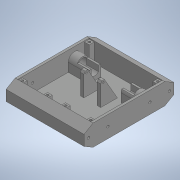
# Autodesk Inventor part: HexBody
Saved by Autodesk Inventor 2020 (Build 240168000, 168)
## iProperties
Created: 2023-12-19
Part Number: HexBody
Material: H TPU
Document SubType Name: Modeling
Designer: smz3rm
Density: 0.941117 g/cm^3
Appearance: Generic(1)
Mass: 192.809 g
Surface Area: 757.089 cm^2
Volume: 204.872 cm^3
BaseThickness: 3.000 mm
TopThickness: 1.778 mm
SideThickness: 4.000 mm
BodyWidth: 130.000 mm
BodyLength: 150.000 mm
BodyHeight: 35.000 mm
DriveMotorHeight: 17.500 mm
WheelWidth: 13.000 mm
WheelGrooveWidth: 4.000 mm
WheelGrooveDia: 15.400 mm
WheelDia: 38.500 mm
WheelPulleyDia: 2.000 mm
M3ScrewInsertBrim: 8.000 mm
M3ScrewDia: 3.100 mm
M3ScrewHeadDia: 6.100 mm
M3ScrewInsertDia: 4.000 mm
M3ScrewInsertDepth: 7.000 mm
DriveMotorOffset: 40.000 mm
DriveMotorHoleDia: 4.200 mm
M3ScrewHeadDepth: 2.200 mm
M3ScrewHeadTaper: -32.50 deg
WheeGuardlSlotWidth: 20.000 mm
WheelGuardScrewOffset: 7.000 mm
FlipperLength: 90.000 mm
FlipperThickness: 4.000 mm
FlipperWidth: 20.000 mm
WheelSpokes: 5.000 ul
FlipperRodDia: 2.000 mm
Author: smz3rm
Autodesk Inventor part; units mm, degrees
ref_plane "XZ Plane" through (0, 0, 0) normal (0, 1, 0) x (-1, 0, 0)
ref_plane "XY Plane" through (0, 0, 0) normal (0, 0, 1) x (1, 0, 0)
sketch "Sketch1" plane through (0, 0, 0) normal (1, 0, 0) x (0, 1, 0)
  line L0 (-17.5, 75) -> (17.5, 75)
  line L1 (17.5, 75) -> (17.5, -75)
  line L2 (17.5, -75) -> (-17.5, -75)
  line L3 (-17.5, -75) -> (-17.5, 75)
  line L4 (-17.5, 75) -> (17.5, -75) construction
  line L5 (17.5, 75) -> (-17.5, -75) construction
  line L6 (-24.5, 0) -> (24.5, 0) projected
  line L7 (0, -105) -> (0, 105) projected
  line L8 (8.75, -75) -> (-8.75, -75)
  line L9 (-8.75, -75) -> (-17.5, -59.8446)
  line L10 (-17.5, -59.8446) -> (-8.75, -44.6891)
  line L11 (-8.75, -44.6891) -> (8.75, -44.6891)
  line L12 (8.75, -44.6891) -> (17.5, -59.8446)
  line L13 (17.5, -59.8446) -> (8.75, -75)
  line L14 (-8.75, 75) -> (-17.5, 59.8446)
  line L15 (17.5, 59.8446) -> (8.75, 75)
  point P0 (0, 0)
  point P1 (0, -59.8446)
  dimension "d0" = 35
  dimension "d1" = 150
  dimension "d25" = 15.1554
  constraints: 28 end point, 4 point on line, 4 symmetric about line, 2 midpoint, 2 parallel, 1 horizontal, 1 perpendicular, 13 other
  measures "d0" distance of L1.end L2.end
  measures "d1" distance of L0.end L1.end
  measures "d25" distance from line of point (0, -59.845) L2
extrude "Extrusion1" add sketch "Sketch1" along normal mid plane 130 contours L0 L7 L6 L3 L14 | L0 L15 L1 L6 L7 | L6 L7 L11 L10 L3 | L6 L1 L12 L11 L7 | L10 L11 L7 L2 L9 | L11 L12 L13 L2 L7
sketch "Sketch2" plane through (-65, 17.5, 60.2776) normal (0, 1, 0) x (1, 0, 0)
  line L0 (130, 120.1221) -> (130, 0.433) projected
  line L1 (0, 0.433) -> (0, 120.1221) projected
  line L2 (126, 120.1221) -> (4, 120.1221)
  line L3 (4, 120.1221) -> (4, 0.433)
  line L4 (4, 0.433) -> (126, 0.433)
  line L5 (126, 0.433) -> (126, 120.1221)
  line L6 (126, 120.1221) -> (4, 0.433) construction
  line L7 (4, 120.1221) -> (126, 0.433) construction
  line L8 (0, 0.433) -> (130, 0.433) projected
  line L9 (0, 120.1221) -> (130, 120.1221) projected
  point P0 (65, 60.2776)
  dimension "d4" = 4
  constraints: 12 end point, 2 midpoint, 2 parallel, 1 horizontal, 1 perpendicular, 1 point on line
  measures "d4" distance between parallel lines of L1 L3
extrude "Extrusion2" cut sketch "Sketch2" against normal blind 32 contours L5 L4 L3 L2
sketch "Sketch3" plane through (-65, -14.5, 60.2776) normal (0, 1, 0) x (1, 0, 0)
  line L0 (4, 0.433) -> (4, 120.1221) projected
  line L1 (126, 0.433) -> (4, 0.433) projected
  line L2 (126, 120.1221) -> (126, 0.433) projected
  line L3 (4, 120.1221) -> (126, 120.1221) projected
  line L4 (4, 0.433) -> (4, 120.1221) projected
  line L5 (126, 120.1221) -> (126, 0.433) projected
  line L6 (130, 120.1221) -> (130, 0.433) projected
  line L7 (0, 0.433) -> (0, 120.1221) projected
  line L8 (4, 120.1221) -> (12, 120.1221)
  line L9 (12, 120.1221) -> (12, 112.1221)
  line L10 (12, 112.1221) -> (4, 112.1221)
  line L11 (4, 112.1221) -> (4, 120.1221)
  line L12 (-26, 60.2776) -> (156, 60.2776) projected
  line L13 (65, 165.2776) -> (65, -44.7224) projected
  line L14 (118, 120.1221) -> (118, 112.1221)
  line L15 (118, 112.1221) -> (126, 112.1221)
  line L16 (12, 0.433) -> (12, 8.433)
  line L17 (12, 8.433) -> (4, 8.433)
  line L18 (118, 0.433) -> (118, 8.433)
  line L19 (118, 8.433) -> (126, 8.433)
  line L20 (0, 120.1221) -> (4, 120.1221) projected
  line L21 (0, 0.433) -> (4, 0.433) projected
  line L22 (126, 0.433) -> (130, 0.433) projected
  line L23 (126, 120.1221) -> (130, 120.1221) projected
  point P0 (65, 60.2776)
  point P1 (12, 0.433)
  point P2 (4, 112.1221)
  point P3 (126, 8.433)
  point P4 (118, 0.433)
  dimension "d8" = 8
  constraints: 20 end point, 9 symmetric about line, 2 parallel, 2 perpendicular, 1 horizontal
  measures "d8" distance of L9.end L10.end
extrude "Extrusion3" add sketch "Sketch3" along normal blind 30.222 contours L0 L17 L16 L1 | L0 L3 L9 L10 | L18 L19 L2 L1 | L15 L14 L3 L2
sketch "Sketch4" plane through (-61, 17.5, 59.8446) normal (1, 0, 0) x (0, 0, -1)
  circle A0 centre (94.8446, -17.5) radius 8.25
  line L0 (119.6891, -35) -> (0, -35) projected
  line L1 (134.8446, -8.75) -> (134.8446, -26.25) projected
  circle A1 centre (94.8446, -17.5) radius 10.25
  line L2 (84.5946, -17.5) -> (84.5946, -32)
  line L3 (8, -32) -> (111.6891, -32) projected
  line L4 (105.0946, -17.5) -> (105.0946, -32)
  point P0 (59.8446, -17.5)
  dimension "d12" = 16.5
  dimension "d13" = 17.5
  dimension "d14" = 40
  dimension "d15" = 2
  constraints: 4 end point, 2 centre point, 2 point on circle, 2 point on line, 2 tangent, 2 vertical, 1 coincident
  measures "d12" diameter of A0
  measures "d13" distance from line of L0 A0.centre
  measures "d14" distance from line of L1 A0.centre
  measures "d15" radial gap between concentric circles of A0 A1
extrude "Extrusion4" add sketch "Sketch4" along normal blind 14
sketch "Sketch5" plane through (-47, 17.5, 59.8446) normal (1, 0, 0) x (0, 0, -1)
  circle A0 centre (94.8446, -17.5) radius 8.25 projected
  circle A1 centre (94.8446, -17.5) radius 7.75
  line L0 (105.0946, -32) -> (105.0946, -17.5) projected
  arc A2 (105.0946, -17.5) -> (84.5946, -17.5) centre (94.8446, -17.5) ccw projected
  line L1 (84.5946, -17.5) -> (84.5946, -32) projected
  line L2 (105.0946, -32) -> (84.5946, -32) projected
  circle A3 centre (94.8446, -17.5) radius 8.25 projected
  line L3 (88.7446, -12.7196) -> (85.7776, -12.7196)
  arc A4 (105.0946, -17.5) -> (84.5946, -17.5) centre (94.8446, -17.5) ccw projected
  line L4 (88.7446, -12.7196) -> (88.7446, -32)
  line L5 (105.0946, -32) -> (84.5946, -32) projected
  line L6 (100.9446, -12.7196) -> (103.9115, -12.7196)
  line L7 (100.9446, -12.7196) -> (100.9446, -32)
  point P0 (59.8446, -17.5)
  point P1 (88.7446, -22.2804)
  point P2 (85.7776, -12.7196)
  point P3 (100.9446, -22.2804)
  dimension "d18" = 15.5
  dimension "d19" = 12.2
  constraints: 8 end point, 4 point on circle, 2 horizontal, 2 perpendicular, 2 point on line, 1 centre point, 1 coincident, 1 parallel
  measures "d18" diameter of A1
  measures "d19" distance between parallel lines of L7 L4
extrude "Extrusion5" add sketch "Sketch5" along normal blind 20 contours A0 L7 A1 L6 | A0 L6 A2 L0 L2 L7 | L7 L2 L4 A0 | A0 L4 A1 L7 | L3 A1 L4 A0 | A0 L4 L2 L1 A2 L3 | A1 L7 | L4 A1
sketch "Sketch6" plane through (-61, 0, -35) normal (1, 0, 0) x (0, 0, -1)
  circle A0 centre (0, 0) radius 2.1
  point P0 (-35, 0)
  dimension "d22" = 4.2
  constraints: 1 centre point
  measures "d22" diameter of A0
extrude "Extrusion6" cut sketch "Sketch6" against normal through all
mirror "Mirror1" about plane through (0, 0, 0) normal (1, 0, 0) of "Extrusion4", "Extrusion5", "Extrusion6"
sketch "Sketch7" plane through (-65, 0, 0) normal (-1, 0, 0) x (0, 0, 1)
  line L0 (-105, 0) -> (105, 0) projected
  circle A0 centre (35, 0) radius 2
  line L1 (75, -8.75) -> (75, 8.75) projected
  point P0 (0, 0)
  dimension "d26" = 4
  dimension "d27" = 40
  constraints: 1 centre point, 1 point on line
  measures "d26" diameter of A0
  measures "d27" distance from line of L1 A0.centre
extrude "Extrusion7" cut sketch "Sketch7" against normal up to surface (4 mm away)
mirror "Mirror2" about plane through (0, 0, 0) normal (1, 0, 0) of "Extrusion7"
sketch "Sketch9" plane through (-65, 0, 0) normal (-1, 0, 0) x (0, 0, 1)
  line L0 (-59.8446, 17.5) -> (-59.8446, 15.722) projected
  line L1 (-59.8446, -17.5) -> (-59.8446, 17.5)
  line L2 (-75, -8.75) -> (-75, 8.75) projected
  line L3 (-75, 0) -> (-59.8446, 0)
  line L4 (-59.8446, -14.5) -> (-59.8446, 15.722) projected
  circle A0 centre (-67.4223, 0) radius 2
  line L5 (0, -24.5) -> (0, 24.5) projected
  circle A1 centre (67.4223, 0) radius 2
  point P0 (0, 0)
  dimension "d30" = 4
  constraints: 4 end point, 2 centre point, 2 midpoint, 1 perpendicular, 1 point on line, 1 symmetric about line, 1 vertical, 1 other
  measures "d30" diameter of A0
extrude "Extrusion8" cut sketch "Sketch9" against normal blind 7
mirror "Mirror3" about plane through (0, 0, 0) normal (1, 0, 0) of "Extrusion8"
ref_plane "Work Plane1" through (11, 0, 0) normal (1, 0, 0) x (0, 1, 0)
sketch "Sketch10" plane through (11, 0, 0) normal (1, 0, 0) x (0, 1, 0)
  line L0 (-14.5, 51.8446) -> (-14.5, -24.75) projected
  line L1 (-14.5, -0.9008) -> (23.05, -0.9008)
  line L2 (23.05, -0.9008) -> (23.05, -7.0496)
  line L3 (23.05, -7.0496) -> (-14.5, -28.7291)
  circle A0 centre (19.5, -5) radius 1.55
  line L4 (-8.75, -75) -> (8.75, -75) projected
  line L5 (17.5, -59.8446) -> (17.5, 59.8446) projected
  line L6 (-14.5, -24.75) -> (-14.5, -45.25) projected
  line L7 (-14.5, -24.75) -> (-14.5, 51.8446) projected
  line L8 (23.05, -7.0496) -> (19.5, -9.0992)
  line L9 (19.5, -9.0992) -> (15.95, -7.0496)
  line L10 (15.95, -7.0496) -> (15.95, -2.9504)
  line L11 (15.95, -2.9504) -> (19.5, -0.9008)
  line L12 (19.5, -0.9008) -> (23.05, -2.9504)
  line L13 (23.05, -2.9504) -> (23.05, -7.0496)
  point P0 (0, 0)
  point P1 (21.05, -5)
  point P2 (17.5, -10.2539)
  point P3 (17.5, -0.9008)
  dimension "d34" = 3.1
  dimension "d38" = 70
  dimension "d40" = 1.55
  dimension "d41" = 2
  dimension "d44" = 60
  dimension "d45" = 2
  constraints: 18 end point, 4 point on line, 1 coincident, 1 collinear, 1 horizontal, 1 horizontal alignment, 1 perpendicular, 15 other
  measures "d38" distance from line of L4 point (19.5, -5)
  measures "d40" distance of point (19.5, -5) point (21.05, -5)
  measures "d41" distance from line of L5 point (19.5, -5)
  measures "d44" angle of L0 L3
  measures "d45" distance from line of L13 point (21.05, -5)
extrude "Extrusion9" add sketch "Sketch10" along normal blind 6 contours L1 L5 L11 L10 L9 L3 L6 L0 | L1 L11 L5 | L12 L2 L3 L9 L5 L11 | L5 L9 L10 L11 | L5 L9 L3
mirror "Mirror4" about plane through (0, 0, 0) normal (1, 0, 0) of "Extrusion9"
sketch "Sketch12" plane through (-65, -14.5, 60.2776) normal (0, 1, 0) x (1, 0, 0)
  line L0 (48, 89.0067) -> (54, 89.0067) projected
  line L1 (54, 89.0067) -> (54, 61.1784) projected
  line L2 (54, 61.1784) -> (48, 61.1784) projected
  line L3 (48, 61.1784) -> (48, 89.0067) projected
  line L4 (76, 89.0067) -> (82, 89.0067) projected
  line L5 (82, 89.0067) -> (82, 61.1784) projected
  line L6 (82, 61.1784) -> (76, 61.1784) projected
  line L7 (76, 61.1784) -> (76, 89.0067) projected
  line L8 (126, 85.0276) -> (92, 85.0276) projected
  line L9 (92, 85.0276) -> (92, 105.5276) projected
  line L10 (92, 105.5276) -> (126, 105.5276) projected
  line L11 (126, 112.1221) -> (126, 105.5276) projected
  line L12 (126, 112.1221) -> (118, 112.1221) projected
  line L13 (118, 112.1221) -> (118, 120.1221) projected
  line L14 (12, 120.1221) -> (118, 120.1221) projected
  line L15 (12, 120.1221) -> (12, 112.1221) projected
  line L16 (12, 112.1221) -> (4, 112.1221) projected
  line L17 (4, 105.5276) -> (4, 112.1221) projected
  line L18 (4, 105.5276) -> (38, 105.5276) projected
  line L19 (38, 105.5276) -> (38, 85.0276) projected
  line L20 (38, 85.0276) -> (4, 85.0276) projected
  line L21 (4, 8.433) -> (4, 85.0276) projected
  line L22 (4, 8.433) -> (12, 8.433) projected
  line L23 (12, 8.433) -> (12, 0.433) projected
  line L24 (118, 0.433) -> (12, 0.433) projected
  line L25 (118, 0.433) -> (118, 8.433) projected
  line L26 (118, 8.433) -> (126, 8.433) projected
  line L27 (126, 85.0276) -> (126, 8.433) projected
  line L28 (54, 61.1784) -> (48, 61.1784) projected
  line L29 (54, 61.1784) -> (48, 61.1784) projected
  line L30 (82, 61.1784) -> (76, 61.1784) projected
  line L31 (76, 61.1784) -> (82, 61.1784) projected
  line L32 (118, 0.433) -> (12, 0.433) projected
  line L33 (54, 0.433) -> (46, 0.433)
  line L34 (46, 0.433) -> (46, 8.433)
  line L35 (46, 8.433) -> (54, 8.433)
  line L36 (54, 8.433) -> (54, 0.433)
  line L37 (65, 165.2776) -> (65, -44.7224) projected
  line L38 (84, 0.433) -> (84, 8.433)
  line L39 (84, 8.433) -> (76, 8.433)
  line L40 (76, 8.433) -> (76, 0.433)
  point P0 (65, 60.2776)
  dimension "d46" = 8
  constraints: 14 end point, 4 symmetric about line, 2 parallel, 2 perpendicular, 1 collinear, 1 horizontal, 1 point on line
  measures "d46" distance of L34.end L35.end
extrude "Extrusion10" add sketch "Sketch12" along normal blind 30.222 contours L24 L40 L39 L38 | L24 L34 L35 L36
sketch "Sketch13" plane through (-65, 15.722, 60.2776) normal (0, 1, 0) x (1, 0, 0)
  line L0 (4, 112.1221) -> (4, 120.1221) projected
  line L1 (4, 112.1221) -> (12, 112.1221) projected
  line L2 (12, 112.1221) -> (12, 120.1221) projected
  line L3 (4, 120.1221) -> (12, 120.1221) projected
  line L4 (118, 120.1221) -> (126, 120.1221) projected
  line L5 (118, 120.1221) -> (118, 112.1221) projected
  line L6 (118, 112.1221) -> (126, 112.1221) projected
  line L7 (126, 120.1221) -> (126, 112.1221) projected
  line L8 (126, 8.433) -> (126, 0.433) projected
  line L9 (126, 8.433) -> (118, 8.433) projected
  line L10 (118, 8.433) -> (118, 0.433) projected
  line L11 (126, 0.433) -> (118, 0.433) projected
  line L12 (84, 0.433) -> (76, 0.433) projected
  line L13 (84, 0.433) -> (84, 8.433) projected
  line L14 (84, 8.433) -> (76, 8.433) projected
  line L15 (76, 8.433) -> (76, 0.433) projected
  line L16 (54, 0.433) -> (54, 8.433) projected
  line L17 (54, 8.433) -> (46, 8.433) projected
  line L18 (46, 8.433) -> (46, 0.433) projected
  line L19 (54, 0.433) -> (46, 0.433) projected
  line L20 (12, 0.433) -> (4, 0.433) projected
  line L21 (12, 0.433) -> (12, 8.433) projected
  line L22 (12, 8.433) -> (4, 8.433) projected
  line L23 (4, 0.433) -> (4, 8.433) projected
  line L24 (4, 120.1221) -> (126, 120.1221) projected
  line L25 (4, 112.1221) -> (12, 112.1221) projected
  line L26 (4, 0.433) -> (4, 120.1221) projected
  line L27 (12, 120.1221) -> (12, 112.1221) projected
  line L28 (8, 120.1221) -> (8, 112.1221)
  line L29 (4, 116.1221) -> (12, 116.1221)
  line L30 (65, 165.2776) -> (65, -44.7224) projected
  line L31 (156, 60.2776) -> (-26, 60.2776) projected
  circle A0 centre (8, 116.1221) radius 2
  circle A1 centre (122, 116.1221) radius 2
  circle A2 centre (8, 4.433) radius 2
  circle A3 centre (122, 4.433) radius 2
  line L32 (50, 8.433) -> (50, 0.433)
  line L33 (46, 0.433) -> (46, 8.433) projected
  line L34 (46, 4.433) -> (54, 4.433)
  line L35 (54, 8.433) -> (54, 0.433) projected
  circle A4 centre (50, 4.433) radius 2
  circle A5 centre (80, 4.433) radius 2
  point P0 (65, 60.2776)
  dimension "d51" = 4
  dimension "d52" = 4
  constraints: 8 end point, 8 midpoint, 6 centre point, 4 symmetric about line, 2 point on line, 1 parallel, 1 perpendicular, 4 other
  measures "d51" diameter of A0
  measures "d52" diameter of A4
extrude "Extrusion11" cut sketch "Sketch13" against normal blind 7 contours A0 L28 L29 | L29 L28 A0 | L28 L29 A0 | L28 A0 L29 | A4 L32 L34 | L34 L32 A4 | A4 L34 L32 | L34 A4 L32 | A1 | A2 | A3 | A5
equation "\"d0\" = BodyHeight"
equation "\"d1\" = BodyLength"
equation "\"d2\" = BodyWidth"
equation "\"d4\" = SideThickness"
equation "\"d5\" = BodyHeight - BaseThickness"
equation "\"d8\" = M3ScrewInsertBrim"
equation "\"d10\" = -BaseThickness + BodyHeight - TopThickness"
equation "\"d13\" = DriveMotorHeight"
equation "\"d14\" = DriveMotorOffset"
equation "\"d22\" = DriveMotorHoleDia"
equation "\"d26\" = M3ScrewInsertDia"
equation "\"d27\" = DriveMotorOffset"
equation "\"d30\" = M3ScrewInsertDia"
equation "\"d31\" = M3ScrewInsertDepth"
equation "\"d34\" = M3ScrewDia"
equation "\"d38\" = FlipperMountOffset"
equation "\"d40\" = 0.5 * d34"
equation "\"d41\" = 0.5 * FlipperThickness"
equation "\"d42\" = FlipperMountThickness"
equation "\"d46\" = M3ScrewInsertBrim"
equation "\"d48\" = -BaseThickness + BodyHeight - TopThickness"
equation "\"d51\" = M3ScrewInsertDia"
equation "\"d52\" = M3ScrewInsertDia"
equation "\"d53\" = M3ScrewInsertDepth"
equation "\"BaseThickness\" = 3"
equation "\"TopThickness\" = 1.778"
equation "\"SideThickness\" = 4"
equation "\"BodyWidth\" = 130"
equation "\"BodyLength\" = 150"
equation "\"BodyHeight\" = 35"
equation "\"DriveMotorHeight\" = 0.5 * BodyHeight"
equation "\"WheelWidth\" = 13"
equation "\"WheelGrooveWidth\" = 4"
equation "\"WheelGrooveDia\" = 0.4 * WheelDia"
equation "\"WheelPulleyDia\" = 2"
equation "\"M3ScrewInsertBrim\" = 8"
equation "\"M3ScrewDia\" = 3.1"
equation "\"M3ScrewHeadDia\" = 6.1"
equation "\"M3ScrewInsertDia\" = 4"
equation "\"M3ScrewInsertDepth\" = 7"
equation "\"DriveMotorOffset\" = 40"
equation "\"DriveMotorHoleDia\" = 4.2"
equation "\"M3ScrewHeadDepth\" = 2.2"
equation "\"M3ScrewHeadTaper\" = -32.5deg"
equation "\"WheelGuardScrewOffset\" = 7"
equation "\"FlipperLength\" = 90"
equation "\"FlipperThickness\" = 4"
equation "\"FlipperWidth\" = 20"
equation "\"WheelSpokes\" = 5"
equation "\"FlipperRodDia\" = 2"
equation "\"FlipperMountOffset\" = 70"
equation "\"FlipperMountThickness\" = 6"
equation "\"WheelDia\" = 38.5"
body "Solid1"
